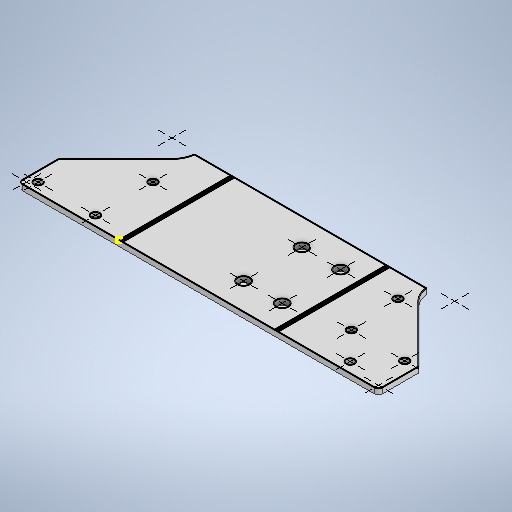
# Autodesk Inventor part: axis_21_bottom_frame
Saved by Autodesk Inventor 2026.1 (Build 301233000, 233)
## iProperties
Created: 2025-08-22
Part Number: axis_21_bottom_frame
Material: Generic
Document SubType Name: Modeling
Designer: LG
Density: 1 g/cm^3
Appearance: Default
Author: LG
Autodesk Inventor part; units mm, degrees
ref_plane "YZ Plane" through (0, 0, 0) normal (1, 0, 0) x (0, 1, 0)
ref_plane "XZ Plane" through (0, 0, 0) normal (0, 1, 0) x (-1, 0, 0)
ref_plane "XY Plane" through (0, 0, 0) normal (0, 0, 1) x (1, 0, 0)
sketch "Sketch1" plane through (0, 0, 0) normal (0, 1, 0) x (-1, 0, 0)
  line L0 (-0.4496, -29.3) -> (-0.4496, 0)
  line L1 (-41.2289, 0) -> (-41.2289, -29.3)
  circle A0 centre (8.735, -17.6) radius 1.05
  circle A1 centre (8.735, -2.5) radius 1.05
  circle A2 centre (23.785, -2.5) radius 1.05
  circle A3 centre (-25.6393, -7) radius 1.55
  circle A4 centre (-35.7793, -7) radius 1.55
  circle A5 centre (-25.6393, -22.3) radius 1.55
  circle A6 centre (-35.7793, -22.3) radius 1.55
  circle A7 centre (-49.9386, -23.2) radius 1.05
  circle A8 centre (-50.9386, -9.98) radius 1.05
  circle A9 centre (-57.9386, -2.68) radius 1.05
  circle A10 centre (-64.9386, -9.98) radius 1.05
  line L2 (11.487, -25.327) -> (26.33, -10.4841)
  line L3 (26.33, -1) -> (26.33, -10.4841)
  line L4 (-68.0086, -10.4841) -> (-53.1656, -25.327)
  line L5 (-68.0086, -10.4841) -> (-68.0086, -1)
  arc A11 (-51.2361, -29.3) -> (-53.1656, -25.327) centre (-57.9386, -30.1) ccw
  line L6 (9.5576, -29.3) -> (-51.2361, -29.3)
  arc A12 (11.487, -25.327) -> (9.5576, -29.3) centre (16.26, -30.1) ccw
  arc A13 (26.33, -1) -> (25.33, 0) centre (25.33, -1) ccw
  line L7 (-67.0086, 0) -> (25.33, 0)
  arc A14 (-67.0086, 0) -> (-68.0086, -1) centre (-67.0086, -1) ccw
  line L8 (-41.6786, -29.3) -> (-41.6786, 0)
  line L9 (-40.7793, 0) -> (-40.7793, -29.3)
  line L10 (-0.8993, -29.3) -> (-0.8993, 0)
  line L11 (0, 0) -> (0, -29.3)
  point P0 (0, 0)
  constraints: 24 end point, 15 centre point, 12 point on line, 11 equal radius, 8 point on circle, 8 vertical, 7 parallel, 6 tangent, 3 perpendicular, 2 horizontal, 55 other
extrude "Extrusion1" add sketch "Sketch1" against normal blind 1.5
body "Solid1"
